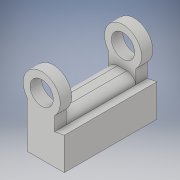
# Autodesk Inventor part: HingeBase1
Saved by Autodesk Inventor 2019 (Build 230136000, 136)
## iProperties
Created: 2019-01-13
Part Number: HingeBase1
Material: Generic
Document SubType Name: Modeling
Designer: Kepler
Density: 1 g/cm^3
Appearance: Default
Mass: 1.46192 g
Surface Area: 10.5158 cm^2
Volume: 1.46192 cm^3
Author: Kepler
Autodesk Inventor part; units mm, degrees
ref_plane "YZ Plane" through (0, 0, 0) normal (1, 0, 0) x (0, 1, 0)
ref_plane "XZ Plane" through (0, 0, 0) normal (0, 1, 0) x (-1, 0, 0)
ref_plane "XY Plane" through (0, 0, 0) normal (0, 0, 1) x (1, 0, 0)
sketch "Sketch1" plane through (0, 0, 0) normal (0, 0, 1) x (1, 0, 0)
  line L0 (0, 0) -> (0, 10)
  line L1 (5.9219, 9.6429) -> (5.9219, 6.6429)
  circle A0 centre (3.1225, 12.5) radius 2.5
  arc A1 (5.9219, 9.6429) -> (0, 10) centre (3.1225, 12.5) ccw
  line L2 (6, 10) -> (0, 10) construction
  line L3 (8, 0) -> (8, 7)
  line L4 (8, 7) -> (5.9219, 6.6429)
  line L5 (0, 0) -> (8, 0)
  dimension "d2" = 8
  dimension "d3" = 5
  dimension "d5" = 10
  dimension "d17" = 7
  dimension "d18" = 3
  dimension "d19" = 8
  constraints: 12 end point, 2 centre point, 2 horizontal, 2 parallel, 2 point on circle, 1 coincident, 1 tangent, 1 vertical
  measures "d2" diameter of A1
  measures "d3" diameter of A0
  measures "d5" distance of L0.start L0.end
  measures "d17" distance of L3.start L3.end
  measures "d18" distance of L1.start L1.end
  measures "d19" distance of L0.start L3.start
extrude "Extrusion1" add sketch "Sketch1" along normal blind 20
sketch "Sketch2" plane through (0, 0, 0) normal (-1, 0, 0) x (0, 0, 1)
  point P0 (0, 0)
sketch "Sketch3" plane through (5.9219, 0, 0) normal (1, 0, 0) x (0, 0, -1)
  line L0 (0, 9.6429) -> (-20, 9.6429) projected
  line L1 (-17.5032, 9.6429) -> (-17.5032, 16.2584)
  line L2 (-17.5032, 16.2584) -> (-2.428, 16.2584)
  line L3 (0, 16.5) -> (-20, 16.5) projected
  line L4 (-2.428, 16.2584) -> (-2.428, 9.6429)
  line L5 (-2.428, 9.6429) -> (-17.5032, 9.6429)
  point P0 (0, 0)
  constraints: 8 end point, 3 perpendicular, 1 parallel, 1 point on line
extrude "Extrusion2" cut sketch "Sketch3" along normal mid plane 20
sketch "Sketch4" plane through (5.9219, 0, 0) normal (1, 0, 0) x (0, 0, -1)
  line L0 (0, 0) -> (-20, 0) projected
  line L1 (0, 0) -> (0, 10) projected
  line L2 (-20, 0) -> (0, 0)
  line L3 (0, 0) -> (0, 6.4437)
  line L4 (0, 6.4437) -> (-20, 6.4437)
  line L5 (-20, 6.4437) -> (-20, 0)
  constraints: 8 end point, 2 parallel, 1 horizontal, 1 perpendicular, 1 point on line
extrude "Extrusion3" add sketch "Sketch4" along normal blind 0.1
sketch "Sketch5" plane through (5.9219, 9.6429, 17.5032) normal (1, 0, 0) x (0, 0, -1)
  line L0 (0, 6.6156) -> (0, 0) projected
  line L1 (0, 6.6156) -> (0, -1.3844)
  line L2 (0, -1.3844) -> (15.0752, -1.3844)
  line L3 (15.0752, 6.6156) -> (15.0752, -1.3844)
  line L4 (0, 6.6156) -> (15.0752, 6.6156)
  point P0 (17.5032, -9.6429)
  dimension "d12" = 8
  dimension "d13" = 15.0752
  constraints: 8 end point, 2 perpendicular, 1 collinear, 1 parallel
  measures "d12" distance of L0.start L1.end
  measures "d13" distance of L0.start L3.start
extrude "Extrusion4" cut sketch "Sketch5" against normal blind 10
fillet "Fillet1" radius 2 1 edges at (5.9219, 8.2584, 9.9656)
fillet "Fillet2" radius 2 1 edges at (0, 8.2584, 9.9656)
sketch "Sketch6" plane through (8, 0, 0) normal (1, 0, 0) x (0, 0, -1)
  line L0 (-2.428, 6.6429) -> (-2.428, 9.6429) projected
  line L1 (-2.428, 9.6429) -> (-17.5032, 9.6429)
  line L2 (-17.5032, 18.1901) -> (-2.428, 18.1901)
  line L3 (0, 9.6429) -> (-2.428, 9.6429) projected
  line L4 (-2.428, 18.1901) -> (-2.428, 9.6429)
  line L5 (-17.5032, 16.2584) -> (-17.5032, 9.6429) projected
  line L6 (-17.5032, 18.1901) -> (-17.5032, 9.6429)
  point P0 (0, 0)
  constraints: 8 end point, 2 perpendicular, 1 collinear, 1 parallel, 1 vertical
extrude "Extrusion5" cut sketch "Sketch6" against normal blind 10
body "Solid1"
